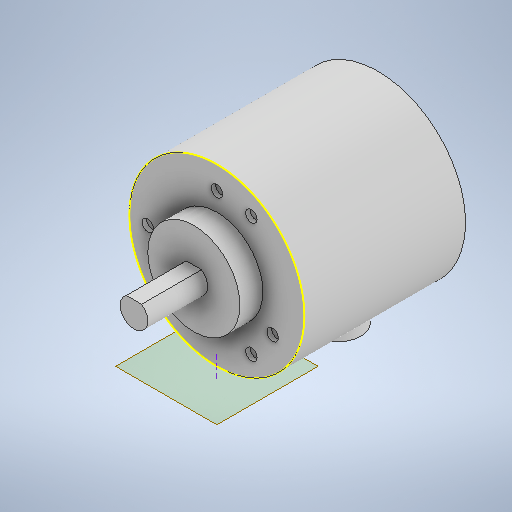
# Autodesk Inventor part: Optical Encoder
Saved by Autodesk Inventor 2025 (Build 290162000, 162)
## iProperties
Created: 2026-05-26
Part Number: Optical Encoder
Material: Generic
Document SubType Name: Sheet Metal
Designer: matot
Density: 1 g/cm^3
Sheet Metal Rule: Default_mm
Appearance: Default
Author: matot
Autodesk Inventor part; units mm, degrees
ref_plane "YZ Plane" through (0, 0, 0) normal (1, 0, 0) x (0, 1, 0)
ref_plane "XZ Plane" through (0, 0, 0) normal (0, 1, 0) x (-1, 0, 0)
ref_plane "XY Plane" through (0, 0, 0) normal (0, 0, 1) x (1, 0, 0)
sketch "Sketch1" plane through (0, 0, 0) normal (0, 0, 1) x (1, 0, 0)
  circle A0 centre (0, 0) radius 3
  line L0 (0, 3) -> (0, 3)
  line L1 (-1.6583, 2.5) -> (1.6583, 2.5)
  line L2 (1.6583, 2.5) -> (1.6583, 4.0802)
  line L3 (-1.6583, 4.0802) -> (-1.6583, 2.5)
  point P0 (0, 2.5)
  dimension "d0" = 6
  dimension "d3" = 2.5
  dimension "d4" = 0
  dimension "d5" = 0.5
  constraints: 8 end point, 3 point on circle, 2 horizontal, 2 midpoint, 1 centre point, 1 coincident, 1 parallel, 1 perpendicular
  measures "d0" diameter of A0
  measures "d3" distance of point (0, 0) point (0, 2.5)
  measures "d4" horizontal distance of point (0, 0) point (0, 2.5)
  measures "d5" distance of point (0, 2.5) point (0, 3)
extrude "Extrusion1" add sketch "Sketch1" against normal blind 13 contours A0 L1 picked at (0.1141, 0.6732)
sketch "Sketch2" plane through (0, 0, -13) normal (0, 0, -1) x (-1, 0, 0)
  circle A0 centre (0, 0) radius 10
  dimension "d8" = 20
  constraints: 1 centre point, 1 coincident
  measures "d8" diameter of A0
extrude "Extrusion2" add sketch "Sketch2" along normal blind 5
sketch "Sketch3" plane through (0, 0, -18) normal (0, 0, -1) x (-1, 0, 0)
  circle A0 centre (0, 0) radius 19
  dimension "d11" = 38
  constraints: 1 centre point, 1 coincident
  measures "d11" diameter of A0
extrude "Extrusion3" add sketch "Sketch3" along normal blind 35
sketch "Sketch4" plane through (0, 0, -18) normal (0, 0, 1) x (1, 0, 0)
  arc A0 (-1.6583, 2.5) -> (1.6583, 2.5) centre (0, 0) ccw projected
  circle A1 centre (0, 0) radius 14
  circle A2 centre (0, 14) radius 1.25
  circle A3 centre (-12.1244, -7) radius 1.25
  circle A4 centre (12.1244, -7) radius 1.25
  circle A5 centre (0, 0) radius 15
  circle A6 centre (7.5, 12.9904) radius 1.25
  circle A7 centre (-15, 0) radius 1.25
  circle A8 centre (7.5, -12.9904) radius 1.25
  dimension "d14" = 28
  dimension "d20" = 30
  dimension "d15" = 2.5
  dimension "d18" = 360
  dimension "d21" = 2.5
  dimension "d22" = 30
  dimension "d25" = 360
  constraints: 6 centre point, 2 coincident, 1 vertical alignment, 19 other
  measures "d15" diameter of A2
  measures "d21" diameter of A6
extrude "Extrusion4" cut sketch "Sketch4" against normal blind 1 contours A6 A1 | A1 A6 A5 | A4 A5 A1 | A1 A4 | A5 A6 | A4 A5 | A2 A1 | A1 A2 A5 | A8 A5 A1 | A1 A8 | A5 A2 | A8 A5 | A7 A1 | A1 A7 A5 | A3 A5 A1 | A1 A3 | A5 A7 | A3 A5
sketch "Sketch5" plane through (0, 0, -18) normal (0, 0, 1) x (1, 0, 0)
  circle A0 centre (0, 0) radius 19 projected
  point P0 (0, -19)
  constraints: 1 vertical alignment, 1 other
ref_plane "Work Plane1" through (0, -19, -18) normal (0, -1, 0) x (1, 0, 0)
sketch "Sketch6" plane through (0, -19, -18) normal (0, -1, 0) x (1, 0, 0)
  circle A0 centre (0, -26.2836) radius 5
  point P0 (0, 18)
  dimension "d29" = 10
  constraints: 1 centre point
  measures "d29" diameter of A0
extrude "Extrusion5" add sketch "Sketch6" along normal blind 5 and the other way blind 0.7
equation "\"BendRadius\" = Thickness"
equation "\"BendReliefWidth\" = Thickness"
equation "\"BendReliefDepth\" = 0.5 * Thickness"
equation "\"CornerReliefSize\" = 4 * Thickness"
equation "\"MinimumRemnant\" = 2 * Thickness"
equation "\"TransitionRadius\" = BendRadius"
equation "\"JacobiRadiusSize\" = BendRadius"
equation "\"GapSize\" = Thickness"
equation "\"Thickness\" = 0.5"
body "Solid1"
